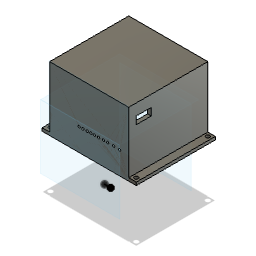
3d Packing (Autodesk Fusion 360 design; units mm, degrees)
Autodesk Fusion 360 part; units mm, degrees
box "BoxPrimitive1" add length 105 width 105 height 5 placed x (0, 0, -1) y (-1, 0, 0) z (0, 1, 0) at (0, 0, 0)
sketch "Sketch2" plane through (0, 5, 0) normal (0, 1, 0) x (-1, 0, 0)
  line L0 (0, -105) -> (105, -105)
  line L1 (105, -105) -> (105, 0)
  line L2 (105, 0) -> (0, 0)
  line L3 (0, 0) -> (0, -105)
sketch "Sketch3" plane through (0, 0, 0) normal (0, -1, 0) x (1, 0, 0)
  line L0 (-105, -105) -> (0, -105)
  line L1 (0, -105) -> (0, 0)
  line L2 (0, 0) -> (-105, 0)
  line L3 (-105, 0) -> (-105, -105)
  line L4 (0, 0) -> (-5, 0)
  line L5 (-5, 0) -> (-5, -105)
  line L6 (-5, -105) -> (0, -105)
  line L7 (0, -105) -> (0, 0)
  line L8 (-105, 0) -> (-100, 0)
  line L9 (-100, 0) -> (-100, -105)
  line L10 (-100, -105) -> (-105, -105)
  line L11 (-105, -105) -> (-105, 0)
  dimension "d6" = 5
  dimension "d7" = 105
  dimension "d8" = 5
  dimension "d9" = 105
  constraint horizontal L4
  constraint vertical L5
  constraint horizontal L6
  constraint vertical L7
  constraint coincident L1.end L2.start
  constraint horizontal L8
  constraint vertical L9
  constraint horizontal L10
  constraint vertical L11
  constraint coincident L2.end L3.start
  measures "d6" distance of L1.end L4.end
  measures "d7" distance of L1.end L0.end
  measures "d8" distance of L2.end L8.end
  measures "d9" distance of L2.end L0.start
extrude "Extrude1" add sketch "Sketch3" along normal blind 100 contours L0 L1 L2 L4 L5 L6 L7
sketch "Sketch4" plane through (0, 0, 0) normal (0, -1, 0) x (1, 0, 0)
  line L0 (-5, -105) -> (-5, 0)
  line L1 (-5, 0) -> (-105, 0)
  line L2 (-105, 0) -> (-105, -105)
  line L3 (-105, -105) -> (-5, -105)
  line L4 (-105, 0) -> (-100, 0)
  line L5 (-100, 0) -> (-100, -105)
  line L6 (-100, -105) -> (-105, -105)
  line L7 (-105, -105) -> (-105, 0)
  dimension "d12" = 5
  constraint horizontal L4
  constraint vertical L5
  constraint horizontal L6
  constraint vertical L7
  constraint coincident L1.end L2.start
  measures "d12" distance of L1.end L4.end
extrude "Extrude2" add sketch "Sketch4" along normal blind 100 contours L1 L2 L3 L4 L5 L6 L7
sketch "Sketch5" plane through (0, 0, 0) normal (1, 0, 0) x (0, 0, -1)
  line L0 (0, 5) -> (0, -100)
  line L1 (0, -100) -> (105, -100)
  line L2 (105, -100) -> (105, 5)
  line L3 (105, 5) -> (0, 5)
  line L4 (10, -10) -> (30, -10)
  line L5 (30, -10) -> (30, -20)
  line L6 (30, -20) -> (10, -20)
  line L7 (10, -20) -> (10, -10)
  dimension "d15" = 20
  dimension "d16" = 10
  constraint horizontal L4
  constraint vertical L5
  constraint horizontal L6
  constraint vertical L7
  measures "d15" distance of L4.start L4.end
  measures "d16" distance of L4.start L6.end
extrude "Extrude3" cut sketch "Sketch5" against normal blind 5 contours L4 L5 L6 L7
sketch "Sketch6" plane through (0, 0, 0) normal (0, -1, 0) x (1, 0, 0)
  line L0 (-100, 0) -> (-100, -105)
  line L1 (-100, -105) -> (-5, -105)
  line L2 (-5, -105) -> (-5, 0)
  line L3 (-5, 0) -> (-100, 0)
  line L4 (-5, 0) -> (-100, 0)
  line L5 (-100, 0) -> (-100, -5)
  line L6 (-100, -5) -> (-5, -5)
  line L7 (-5, -5) -> (-5, 0)
  dimension "d19" = 5
  constraint horizontal L4
  constraint vertical L5
  constraint horizontal L6
  constraint vertical L7
  constraint coincident L2.end L3.start
  measures "d19" distance of L2.end L6.end
extrude "Extrude4" add sketch "Sketch6" along normal blind 100 contours L0 L2 L3 L4 L5 L6 L7
sketch "Sketch7" plane through (0, 0, 0) normal (0, -1, 0) x (1, 0, 0)
  line L0 (-5, -5) -> (-100, -5)
  line L1 (-100, -5) -> (-100, -105)
  line L2 (-100, -105) -> (-5, -105)
  line L3 (-5, -105) -> (-5, -5)
  line L4 (-5, -105) -> (-100, -105)
  line L5 (-100, -105) -> (-100, -100)
  line L6 (-100, -100) -> (-5, -100)
  line L7 (-5, -100) -> (-5, -105)
  constraint horizontal L4
  constraint vertical L5
  constraint horizontal L6
  constraint vertical L7
  constraint coincident L1 L5.end
  constraint coincident L2.end L3.start
extrude "Extrude5" add sketch "Sketch7" along normal blind 100 contours L1 L2 L3 L4 L5 L6 L7
sketch "Sketch8" plane through (0, 0, 0) normal (0, 0, 1) x (1, 0, 0)
  line L0 (-105, 5) -> (-105, -100)
  line L1 (-105, -100) -> (0, -100)
  line L2 (0, -100) -> (0, 5)
  line L3 (0, 5) -> (-105, 5)
  circle A0 centre (-10, -93) radius 0.51
  line L4 (-10, -93) -> (-12.54, -93)
  circle A1 centre (-12.54, -93) radius 0.51
  line L5 (-12.54, -93) -> (-15.08, -93)
  line L6 (-15.08, -93) -> (-17.62, -93)
  circle A2 centre (-15.08, -93) radius 0.51
  circle A3 centre (-17.62, -93) radius 0.51
  line L7 (-17.62, -93) -> (-20.16, -93)
  circle A4 centre (-20.16, -93) radius 0.51
  line L8 (-20.16, -93) -> (-22.7, -93)
  circle A5 centre (-22.7, -93) radius 0.51
  line L9 (-22.7, -93) -> (-25.24, -93)
  line L10 (-25.24, -93) -> (-27.78, -93)
  circle A6 centre (-25.24, -93) radius 0.51
  circle A7 centre (-27.78, -93) radius 0.51
  dimension "d24" = 1.02
  dimension "d25" = 2.54
  dimension "d26" = 1.02
  dimension "d27" = 2.54
  dimension "d28" = 2.54
  dimension "d29" = 1.02
  dimension "d30" = 1.02
  dimension "d31" = 2.54
  dimension "d32" = 1.02
  dimension "d33" = 2.54
  dimension "d34" = 1.02
  dimension "d35" = 2.54
  dimension "d36" = 2.54
  dimension "d37" = 1.02
  dimension "d38" = 1.02
  constraint coincident A0.centre L4.start
  constraint horizontal L4
  constraint coincident L4.end A1.centre
  constraint parallel L4 L5
  constraint parallel L5 L6
  constraint coincident L5.end L6.start
  constraint coincident L6.end A3.centre
  constraint parallel L6 L7
  constraint coincident L7.end A4.centre
  constraint parallel L7 L8
  constraint coincident L8.end A5.centre
  constraint parallel L8 L9
  constraint parallel L9 L10
  constraint coincident L9.end L10.start
  constraint coincident L10.end A7.centre
  measures "d24" diameter of A0
  measures "d25" distance of A0.centre L4.end
  measures "d26" diameter of A1
  measures "d27" distance of L4.end L5.end
  measures "d28" distance of L5.end L6.end
  measures "d29" diameter of A2
  measures "d30" diameter of A3
  measures "d31" distance of L6.end L7.end
  measures "d32" diameter of A4
  measures "d33" distance of L7.end L8.end
  measures "d34" diameter of A5
  measures "d35" distance of L8.end L9.end
  measures "d36" distance of L9.end L10.end
  measures "d37" diameter of A6
  measures "d38" diameter of A7
extrude "Extrude6" cut sketch "Sketch8" against normal blind 5 contours A0
sketch "Sketch9" plane through (0, 0, 0) normal (0, 0, 1) x (1, 0, 0)
  circle A0 centre (-10, -93) radius 0.51
  line L0 (-105, 5) -> (-105, -100)
  line L1 (-105, -100) -> (0, -100)
  line L2 (0, -100) -> (0, 5)
  line L3 (0, 5) -> (-105, 5)
  line L4 (-10, -93) -> (-12.54, -93)
  circle A1 centre (-12.54, -93) radius 0.51
  dimension "d41" = 2.54
  dimension "d42" = 1.02
  constraint coincident A0.centre L4.start
  constraint horizontal L4
  constraint coincident L4.end A1.centre
  measures "d41" distance of A0.centre L4.end
  measures "d42" diameter of A1
extrude "Extrude7" cut sketch "Sketch9" against normal blind 5 contours A1
sketch "Sketch10" plane through (0, 0, 0) normal (0, 0, 1) x (1, 0, 0)
  circle A0 centre (-12.54, -93) radius 0.51
  circle A1 centre (-10, -93) radius 0.51
  line L0 (-105, 5) -> (-105, -100)
  line L1 (-105, -100) -> (0, -100)
  line L2 (0, -100) -> (0, 5)
  line L3 (0, 5) -> (-105, 5)
  line L4 (-12.54, -93) -> (-15.08, -93)
  circle A2 centre (-15.08, -93) radius 0.51
  dimension "d45" = 2.54
  dimension "d46" = 1.02
  constraint coincident A0.centre L4.start
  constraint horizontal L4
  constraint coincident L4.end A2.centre
  measures "d45" distance of A0.centre L4.end
  measures "d46" diameter of A2
extrude "Extrude8" cut sketch "Sketch10" against normal blind 5 contours A2
sketch "Sketch11" plane through (0, 0, -100) normal (0, 0, 1) x (1, 0, 0)
  line L0 (-5, 0) -> (-100, 0)
  line L1 (-100, 0) -> (-100, -100)
  line L2 (-100, -100) -> (-5, -100)
  line L3 (-5, -100) -> (-5, 0)
sketch "Sketch12" plane through (0, 0, 0) normal (0, 0, 1) x (1, 0, 0)
  circle A0 centre (-15.08, -93) radius 0.51
  circle A1 centre (-12.54, -93) radius 0.51
  circle A2 centre (-10, -93) radius 0.51
  line L0 (-105, 5) -> (-105, -100)
  line L1 (-105, -100) -> (0, -100)
  line L2 (0, -100) -> (0, 5)
  line L3 (0, 5) -> (-105, 5)
  line L4 (-15.08, -93) -> (-17.62, -93)
  circle A3 centre (-17.62, -93) radius 0.51
  dimension "d49" = 2.54
  dimension "d50" = 1.02
  constraint coincident A0.centre L4.start
  constraint perpendicular L2 L4
  constraint coincident L4.end A3.centre
  measures "d49" distance of A0.centre L4.end
  measures "d50" diameter of A3
extrude "Extrude9" cut sketch "Sketch12" against normal blind 5 contours A3
sketch "Sketch13" plane through (0, 0, 0) normal (0, 0, 1) x (1, 0, 0)
  circle A0 centre (-17.62, -93) radius 0.51
  circle A1 centre (-15.08, -93) radius 0.51
  circle A2 centre (-12.54, -93) radius 0.51
  circle A3 centre (-10, -93) radius 0.51
  line L0 (-105, 5) -> (-105, -100)
  line L1 (-105, -100) -> (0, -100)
  line L2 (0, -100) -> (0, 5)
  line L3 (0, 5) -> (-105, 5)
  line L4 (-17.62, -93) -> (-20.16, -93)
  circle A4 centre (-20.16, -93) radius 0.51
  dimension "d53" = 2.54
  dimension "d54" = 1.02
  constraint coincident A0.centre L4.start
  constraint horizontal L4
  constraint coincident L4.end A4.centre
  measures "d53" distance of A0.centre L4.end
  measures "d54" diameter of A4
extrude "Extrude10" cut sketch "Sketch13" against normal blind 5 contours A4
sketch "Sketch14" plane through (0, 0, 0) normal (0, 0, 1) x (1, 0, 0)
  circle A0 centre (-20.16, -93) radius 0.51
  circle A1 centre (-17.62, -93) radius 0.51
  circle A2 centre (-15.08, -93) radius 0.51
  circle A3 centre (-12.54, -93) radius 0.51
  circle A4 centre (-10, -93) radius 0.51
  line L0 (-105, 5) -> (-105, -100)
  line L1 (-105, -100) -> (0, -100)
  line L2 (0, -100) -> (0, 5)
  line L3 (0, 5) -> (-105, 5)
  line L4 (-20.16, -93) -> (-22.7, -93)
  circle A5 centre (-22.7, -93) radius 0.51
  dimension "d57" = 2.54
  dimension "d58" = 1.02
  constraint coincident A0.centre L4.start
  constraint horizontal L4
  constraint coincident L4.end A5.centre
  measures "d57" distance of A0.centre L4.end
  measures "d58" diameter of A5
extrude "Extrude11" cut sketch "Sketch14" against normal blind 5 contours A5
sketch "Sketch15" plane through (0, 0, 0) normal (0, 0, 1) x (1, 0, 0)
  circle A0 centre (-22.7, -93) radius 0.51
  circle A1 centre (-20.16, -93) radius 0.51
  circle A2 centre (-17.62, -93) radius 0.51
  circle A3 centre (-15.08, -93) radius 0.51
  circle A4 centre (-12.54, -93) radius 0.51
  circle A5 centre (-10, -93) radius 0.51
  line L0 (-105, 5) -> (-105, -100)
  line L1 (-105, -100) -> (0, -100)
  line L2 (0, -100) -> (0, 5)
  line L3 (0, 5) -> (-105, 5)
  line L4 (-22.7, -93) -> (-25.24, -93)
  circle A6 centre (-25.24, -93) radius 0.51
  dimension "d61" = 2.54
  dimension "d62" = 1.02
  constraint coincident A0.centre L4.start
  constraint horizontal L4
  constraint coincident L4.end A6.centre
  measures "d61" distance of A0.centre L4.end
  measures "d62" diameter of A6
extrude "Extrude12" cut sketch "Sketch15" against normal blind 5 contours A6
sketch "Sketch16" plane through (0, 0, 0) normal (0, 0, 1) x (1, 0, 0)
  circle A0 centre (-25.24, -93) radius 0.51
  circle A1 centre (-22.7, -93) radius 0.51
  circle A2 centre (-20.16, -93) radius 0.51
  circle A3 centre (-17.62, -93) radius 0.51
  circle A4 centre (-15.08, -93) radius 0.51
  circle A5 centre (-12.54, -93) radius 0.51
  circle A6 centre (-10, -93) radius 0.51
  line L0 (-105, 5) -> (-105, -100)
  line L1 (-105, -100) -> (0, -100)
  line L2 (0, -100) -> (0, 5)
  line L3 (0, 5) -> (-105, 5)
  line L4 (-25.24, -93) -> (-27.78, -93)
  circle A7 centre (-27.78, -93) radius 0.51
  dimension "d65" = 2.54
  dimension "d66" = 1.02
  constraint coincident A0.centre L4.start
  constraint horizontal L4
  constraint coincident L4.end A7.centre
  measures "d65" distance of A0.centre L4.end
  measures "d66" diameter of A7
extrude "Extrude13" cut sketch "Sketch16" against normal blind 5 contours A7
extrude "Extrude14" cut 1 faces at (-44.345, -30.8528, -5) along direction (0, 0, 1) blind 5
sketch "Sketch17" plane through (0, 0, 0) normal (0, -1, 0) x (1, 0, 0)
  line L0 (-100, -100) -> (-5, -100)
  line L1 (-5, -100) -> (-5, 0)
  line L2 (-5, 0) -> (-100, 0)
  line L3 (-100, 0) -> (-100, -100)
  line L4 (-26.837, -47.1859) -> (-5, -47.1859)
  line L5 (-5, -47.1859) -> (-5, 0)
  line L6 (-5, 0) -> (-26.837, 0)
  line L7 (-26.837, 0) -> (-26.837, -47.1859)
  line L8 (-5, 0) -> (-100, 0)
  line L9 (-100, 0) -> (-100, -5)
  line L10 (-100, -5) -> (-5, -5)
  line L11 (-5, -5) -> (-5, 0)
  dimension "d71" = 95
  dimension "d72" = 5
  constraint horizontal L4
  constraint vertical L5
  constraint horizontal L6
  constraint vertical L7
  constraint coincident L1.end L2.start
  constraint horizontal L8
  constraint vertical L9
  constraint horizontal L10
  constraint vertical L11
  measures "d71" distance of L1.end L2.end
  measures "d72" distance of L1.end L10.end
extrude "Extrude15" add sketch "Sketch17" along normal blind 100 contours L1 L2 L5 L6 L7 L8 L10 L11
sketch "Sketch18" plane through (0, 0, 0) normal (0, -1, 0) x (1, 0, 0)
  line L0 (-26.837, -5) -> (-26.837, 0)
  line L1 (-26.837, 0) -> (-100, 0)
  line L2 (-100, 0) -> (-100, -100)
  line L3 (-100, -100) -> (-5, -100)
  line L4 (-5, -100) -> (-5, -5)
  line L5 (-5, -5) -> (-26.837, -5)
  line L6 (-26.837, 0) -> (-100, 0)
  line L7 (-100, 0) -> (-100, -5)
  line L8 (-100, -5) -> (-26.837, -5)
  line L9 (-26.837, -5) -> (-26.837, 0)
  dimension "d75" = 5
  constraint horizontal L6
  constraint vertical L7
  constraint horizontal L8
  constraint vertical L9
  constraint coincident L0.end L1.start
  measures "d75" distance of L0.end L0.start
extrude "Extrude16" add sketch "Sketch18" along normal blind 100 contours L0 L1 L2 L6 L7 L8 L9
extrude "Extrude17" cut 1 faces at (-103.3333, -100, -68.3333) along direction (0, 1, 0) blind 20
sketch "Sketch19" plane through (0, 0, 0) normal (0, 0, 1) x (1, 0, 0)
  line L0 (-105, -80) -> (0, -80)
  line L1 (0, -80) -> (0, 5)
  line L2 (0, 5) -> (-105, 5)
  line L3 (-105, 5) -> (-105, -80)
  circle A0 centre (-20, -50) radius 1.5
  line L4 (-20, -50) -> (-28, -50)
  circle A1 centre (-28, -50) radius 1.5
  line L5 (-28, -50) -> (-36, -50)
  circle A2 centre (-36, -50) radius 1.5
  line L6 (-36, -50) -> (-44, -50)
  circle A3 centre (-44, -50) radius 1.5
  line L7 (-44, -50) -> (-52, -50)
  circle A4 centre (-52, -50) radius 1.5
  line L8 (-52, -50) -> (-60, -50)
  circle A5 centre (-60, -50) radius 1.5
  line L9 (-60, -50) -> (-68, -50)
  circle A6 centre (-68, -50) radius 1.5
  line L10 (-68, -50) -> (-76, -50)
  circle A7 centre (-76, -50) radius 1.5
  line L11 (-76, -50) -> (-84, -50)
  circle A8 centre (-84, -50) radius 1.5
  line L12 (-84, -50) -> (-92, -50)
  circle A9 centre (-92, -50) radius 1.5
  line L13 (-20, -50) -> (-12, -50)
  circle A10 centre (-12, -50) radius 1.5
  dimension "d80" = 3
  dimension "d81" = 8
  dimension "d82" = 3
  dimension "d83" = 8
  dimension "d84" = 3
  dimension "d85" = 8
  dimension "d86" = 3
  dimension "d87" = 8
  dimension "d88" = 3
  dimension "d89" = 8
  dimension "d90" = 3
  dimension "d91" = 8
  dimension "d92" = 3
  dimension "d93" = 8
  dimension "d94" = 3
  dimension "d95" = 8
  dimension "d96" = 3
  dimension "d97" = 8
  dimension "d98" = 3
  dimension "d99" = 8
  dimension "d100" = 3
  constraint coincident A0.centre L4.start
  constraint horizontal L4
  constraint coincident L4.end A1.centre
  constraint parallel L4 L5
  constraint coincident L5.end A2.centre
  constraint parallel L5 L6
  constraint coincident L6.end A3.centre
  constraint parallel L6 L7
  constraint coincident L7.end A4.centre
  constraint parallel L7 L8
  constraint coincident L8.end A5.centre
  constraint parallel L8 L9
  constraint coincident L9.end A6.centre
  constraint parallel L9 L10
  constraint coincident L10.end A7.centre
  constraint parallel L10 L11
  constraint coincident L11.end A8.centre
  constraint parallel L11 L12
  constraint coincident L12.end A9.centre
  constraint parallel L4 L13
  constraint coincident L13.end A10.centre
  measures "d80" diameter of A0
  measures "d81" distance of A0.centre L4.end
  measures "d82" diameter of A1
  measures "d83" distance of L4.end L5.end
  measures "d84" diameter of A2
  measures "d85" distance of L5.end L6.end
  measures "d86" diameter of A3
  measures "d87" distance of L6.end L7.end
  measures "d88" diameter of A4
  measures "d89" distance of L7.end L8.end
  measures "d90" diameter of A5
  measures "d91" distance of L8.end L9.end
  measures "d92" diameter of A6
  measures "d93" distance of L9.end L10.end
  measures "d94" diameter of A7
  measures "d95" distance of L10.end L11.end
  measures "d96" diameter of A8
  measures "d97" distance of L11.end L12.end
  measures "d98" diameter of A9
  measures "d99" distance of A0.centre L13.end
  measures "d100" diameter of A10
hole "Hole1" at (-12, -50, 0) direction (0, 0, -1) diameter 3 depth 5 tip angle 118
sketch "Sketch20" plane through (0, 0, 0) normal (0, 0, 1) x (1, 0, 0)
  circle A0 centre (-12, -50) radius 1.5
  line L0 (-105, -80) -> (0, -80)
  line L1 (0, -80) -> (0, 5)
  line L2 (0, 5) -> (-105, 5)
  line L3 (-105, 5) -> (-105, -80)
  line L4 (-12, -50) -> (-20, -50)
  dimension "d104" = 8
  constraint coincident A0.centre L4.start
  constraint horizontal L4
  measures "d104" distance of A0.centre L4.end
move_body "Move1" bodies 1 to x (1, 0, 0) y (0, 1, 0) z (0, 0, 1) at (11.0146, 50.57, 0)
sketch "Sketch21" plane through (0, 0, 0) normal (0, 0, 1) x (1, 0, 0)
  circle A0 centre (-0.9854, 0.57) radius 1.5
  line L0 (-93.9854, -29.43) -> (11.0146, -29.43)
  line L1 (11.0146, -29.43) -> (11.0146, 55.57)
  line L2 (11.0146, 55.57) -> (-93.9854, 55.57)
  line L3 (-93.9854, 55.57) -> (-93.9854, -29.43)
move_body "Move2" bodies 1 to x (1, 0, 0) y (0, 1, 0) z (0, 0, 1) at (0.9697, -0.9697, 0)
sketch "Sketch22" plane through (0, 0, 0) normal (0, 0, 1) x (1, 0, 0)
  line L0 (0, 0) -> (-8, 0)
  dimension "d105" = 8
  constraint coincident L0.start origin
  constraint horizontal L0
  measures "d105" distance of L0.start L0.end
hole "Hole2" at (-8, 0, 0) direction (0, 0, -1) diameter 3 depth 5 tip angle 118
sketch "Sketch23" plane through (0, 0, 0) normal (0, 0, 1) x (1, 0, 0)
sketch "Sketch24" plane through (0, 0, 0) normal (0, 0, 1) x (1, 0, 0)
  line L0 (-8, 0) -> (-16, 0)
  dimension "d109" = 8
  constraint horizontal L0
  measures "d109" distance of L0.start L0.end
hole "Hole3" at (-16, 0, 0) direction (0, 0, -1) diameter 3 depth 5 tip angle 118
hole "Hole4" at (-21.5007, 0.0439, 0) direction (0, 0, -1) diameter 3 depth 5 tip angle 118
hole "Hole5" at (-28.022, -0.0676, 0) direction (0, 0, -1) diameter 3 depth 5 tip angle 118
hole "Hole6" at (-33.54, -0.1233, 0) direction (0, 0, -1) diameter 3 depth 5 tip angle 118
hole "Hole7" at (-38.2777, -0.3091, 0) direction (0, 0, -1) diameter 3 depth 5 tip angle 118
hole "Hole8" at (-43.2569, -0.4577, 0) direction (0, 0, -1) diameter 3 depth 5 tip angle 118
hole "Hole9" at (-48.7934, -0.6621, 0) direction (0, 0, -1) diameter 3 depth 5 tip angle 118
hole "Hole10" at (-53.977, -0.6621, 0) direction (0, 0, -1) diameter 3 depth 5 tip angle 118
sketch "Sketch25" plane through (11.9842, 0, 0) normal (1, 0, 0) x (0, 0, -1)
  line L0 (0, -30.3997) -> (105, -30.3997)
  line L1 (105, -30.3997) -> (105, 54.6003)
  line L2 (105, 54.6003) -> (0, 54.6003)
  line L3 (0, 54.6003) -> (0, -30.3997)
  line L4 (30, 39.6003) -> (30, 29.6003)
  line L5 (30, 29.6003) -> (10, 29.6003)
  line L6 (10, 29.6003) -> (10, 39.6003)
  line L7 (10, 39.6003) -> (30, 39.6003)
  line L8 (0, -30.3997) -> (105, -30.3997)
  line L9 (105, -30.3997) -> (105, -26.3997)
  line L10 (105, -26.3997) -> (0, -26.3997)
  line L11 (0, -26.3997) -> (0, -30.3997)
  dimension "d135" = 4
  constraint horizontal L8
  constraint vertical L9
  constraint horizontal L10
  constraint vertical L11
  constraint coincident L0.start L3.end
  measures "d135" distance of L0.start L10.end
extrude "Extrude18" add sketch "Sketch25" along normal blind 5 contours L0 L1 L3 L8 L9 L10 L11
sketch "Sketch26" plane through (-93.0158, 0, 0) normal (-1, 0, 0) x (0, 0, 1)
  line L0 (-105, -30.3997) -> (0, -30.3997)
  line L1 (0, -30.3997) -> (0, 54.6003)
  line L2 (0, 54.6003) -> (-105, 54.6003)
  line L3 (-105, 54.6003) -> (-105, -30.3997)
  line L4 (0, -30.3997) -> (-105, -30.3997)
  line L5 (-105, -30.3997) -> (-105, -26.3997)
  line L6 (-105, -26.3997) -> (0, -26.3997)
  line L7 (0, -26.3997) -> (0, -30.3997)
  dimension "d138" = 4
  constraint horizontal L4
  constraint vertical L5
  constraint horizontal L6
  constraint vertical L7
  constraint coincident L0.end L1.start
  measures "d138" distance of L0.end L6.end
extrude "Extrude19" add sketch "Sketch26" along normal blind 5 contours L0 L1 L3 L4 L5 L6 L7
extrude "Extrude20" add 1 faces at (-98.0158, -27.733, -70) along direction (-1, 0, 0) blind 5
extrude "Extrude21" add 1 faces at (16.9842, -29.0664, -70) along direction (1, 0, 0) blind 5
sketch "Sketch27" plane through (0, -26.3997, 0) normal (0, 1, 0) x (-1, 0, 0)
  line L0 (-11.9842, -105) -> (-11.9842, 0)
  line L1 (-11.9842, 0) -> (-21.9842, 0)
  line L2 (-21.9842, 0) -> (-21.9842, -105)
  line L3 (-21.9842, -105) -> (-11.9842, -105)
  line L4 (-16.9842, 0) -> (-16.9842, -5)
  circle A0 centre (-16.9842, -5) radius 2.5
  dimension "d145" = 5
  dimension "d146" = 5
  constraint midpoint L1 L4.start
  constraint perpendicular L1 L4
  constraint coincident L4.end A0.centre
  measures "d145" distance of L4.start L4.end
  measures "d146" diameter of A0
extrude "Extrude22" cut sketch "Sketch27" against normal blind 5 contours A0
sketch "Sketch28" plane through (0, -26.3997, 0) normal (0, 1, 0) x (-1, 0, 0)
  circle A0 centre (-16.9842, -5) radius 2.5
  line L0 (-11.9842, -105) -> (-11.9842, 0)
  line L1 (-11.9842, 0) -> (-21.9842, 0)
  line L2 (-21.9842, 0) -> (-21.9842, -105)
  line L3 (-21.9842, -105) -> (-11.9842, -105)
  line L4 (-16.9842, -105) -> (-16.9842, -100)
  circle A1 centre (-16.9842, -100) radius 2.5
  dimension "d149" = 5
  dimension "d150" = 5
  constraint midpoint L3 L4.start
  constraint perpendicular L3 L4
  constraint coincident L4.end A1.centre
  measures "d149" distance of L4.start L4.end
  measures "d150" diameter of A1
extrude "Extrude23" cut sketch "Sketch28" against normal blind 5 contours A1
sketch "Sketch29" plane through (0, 5, 0) normal (0, 1, 0) x (-1, 0, 0)
sketch "Sketch30" plane through (0, -26.3997, 0) normal (0, 1, 0) x (-1, 0, 0)
  line L0 (93.0158, 0) -> (93.0158, -105)
  line L1 (93.0158, -105) -> (103.0158, -105)
  line L2 (103.0158, -105) -> (103.0158, 0)
  line L3 (103.0158, 0) -> (93.0158, 0)
  line L4 (98.0158, 0) -> (98.0158, -6)
  circle A0 centre (98.0158, -6) radius 2.5
  dimension "d153" = 6
  dimension "d154" = 5
  constraint midpoint L3 L4.start
  constraint perpendicular L3 L4
  constraint coincident L4.end A0.centre
  measures "d153" distance of L4.start L4.end
  measures "d154" diameter of A0
extrude "Extrude24" cut sketch "Sketch30" against normal blind 5 contours A0
sketch "Sketch31" plane through (0, -26.3997, 0) normal (0, 1, 0) x (-1, 0, 0)
  circle A0 centre (98.0158, -6) radius 2.5
  line L0 (93.0158, 0) -> (93.0158, -105)
  line L1 (93.0158, -105) -> (103.0158, -105)
  line L2 (103.0158, -105) -> (103.0158, 0)
  line L3 (103.0158, 0) -> (93.0158, 0)
  line L4 (98.0158, -105) -> (98.0158, -100)
  circle A1 centre (98.0158, -100) radius 2.5
  dimension "d157" = 5
  dimension "d158" = 5
  constraint midpoint L1 L4.start
  constraint perpendicular L1 L4
  constraint coincident L4.end A1.centre
  measures "d157" distance of L4.start L4.end
  measures "d158" diameter of A1
extrude "Extrude25" cut sketch "Sketch31" against normal blind 5 contours A1
